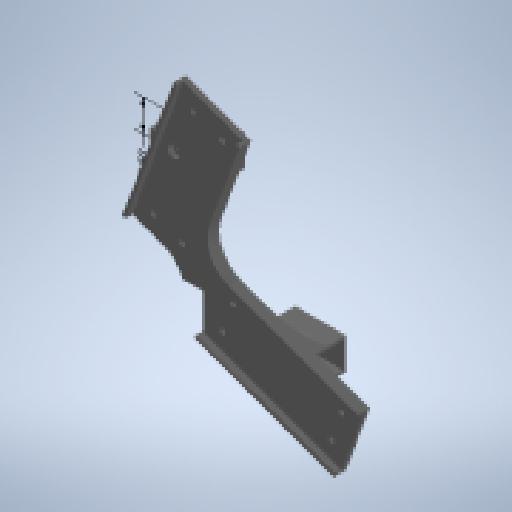
# Autodesk Inventor part: back_base
Saved by Autodesk Inventor 2026.1 (Build 301233020, 233B)
## iProperties
Created: 2026-02-04
Part Number: back_base
Material: 一般
Document SubType Name: Modeling
Designer: hibik
Density: 1 g/cm^3
Appearance: 既定
Author: hibik
Autodesk Inventor part; units mm, degrees
ref_plane "YZ Plane" through (0, 0, 0) normal (1, 0, 0) x (0, 1, 0)
ref_plane "XY Plane" through (0, 0, 0) normal (0, 0, 1) x (1, 0, 0)
sketch "スケッチ1" plane through (0, 0, 0) normal (1, 0, 0) x (0, 1, 0)
  line L0 (-7.75, -7.75) -> (7.75, -7.75)
  line L1 (7.75, -7.75) -> (7.75, 7.75)
  line L2 (7.75, 7.75) -> (-7.75, 7.75)
  line L3 (-7.75, 7.75) -> (-7.75, -7.75)
  line L4 (-7.75, -7.75) -> (7.75, 7.75) construction
  line L5 (7.75, -7.75) -> (-7.75, 7.75) construction
  line L6 (-9.25, 9.25) -> (9.25, 9.25)
  line L7 (9.25, 9.25) -> (9.25, -9.25)
  line L8 (9.25, -9.25) -> (-9.25, -9.25)
  line L9 (-9.25, -9.25) -> (-9.25, 9.25)
  line L10 (-9.25, 9.25) -> (9.25, -9.25) construction
  line L11 (9.25, 9.25) -> (-9.25, -9.25) construction
  point P0 (0, 0)
  dimension "d0" = 15.5
  dimension "d1" = 1.5
  constraints: 24 end point, 4 midpoint, 4 parallel, 3 perpendicular, 2 horizontal, 1 point on line
  measures "d0" distance of L2.end L1.end
  measures "d1" distance between parallel lines of L7 L1
extrude "押し出し1" add sketch "スケッチ1" along normal blind 30
sketch "スケッチ2" plane through (30, 9.25, -9.25) normal (0, 0, -1) x (-1, 0, 0)
  circle A0 centre (20, -9.25) radius 1.6
  line L0 (0, -18.5) -> (0, 0) projected
  point P0 (30, -9.25)
  dimension "d4" = 3.2
  dimension "d6" = 20
  constraints: 1 centre point, 1 horizontal alignment
  measures "d4" diameter of A0
  measures "d6" distance from line of L0 A0.centre
extrude "押し出し2" cut sketch "スケッチ2" against normal through all
sketch "スケッチ4" plane through (0, -9.25, 9.25) normal (0, 0, 1) x (1, 0, 0)
  line L0 (0, 18.5) -> (40, 18.5)
  line L1 (40, 18.5) -> (40, 0)
  line L2 (40, 0) -> (0, 0)
  line L3 (0, 0) -> (0, 18.5)
  circle A0 centre (10, 9.25) radius 1.6 projected
  point P0 (0, 9.25)
  dimension "d13" = 30
  constraints: 8 end point, 2 parallel, 1 horizontal, 1 perpendicular, 1 point on line
  measures "d13" distance from line of L1 A0.centre
extrude "押し出し4" add sketch "スケッチ4" along normal blind 7
sketch "スケッチ5" plane through (0, -9.25, 16.25) normal (0, 0, 1) x (1, 0, 0)
  line L0 (14.0213, 48.5) -> (52.5487, 34.4772)
  line L1 (52.5487, 34.4772) -> (-1.5009, -114.0228)
  line L2 (-1.5009, -114.0228) -> (-40.0283, -100)
  line L3 (-40.0283, -100) -> (14.0213, 48.5)
  line L4 (40, 0) -> (40, 18.5) projected
  line L5 (0, 0) -> (40, 0) projected
  line L6 (40, 18.5) -> (0, 18.5) projected
  line L7 (0, 18.5) -> (0, 0) projected
  point P0 (0, 9.25)
  point P1 (66.3687, 0)
  point P2 (3.1022, 18.5)
  dimension "d16" = 41
  dimension "d17" = 20
  dimension "d23" = 30
  dimension "d24" = 100
  constraints: 8 end point, 2 parallel, 1 perpendicular, 1 point on line
  measures "d16" distance between parallel lines of L1 L3
  measures "d17" angle of L4 L1
  measures "d23" distance from line of L0.start L6
  measures "d24" distance from line of L5 L2.end
extrude "押し出し5" add sketch "スケッチ5" against normal up to surface (7 mm away) contours L0 L1 L4 L6 L3 | L6 L4 L5 L7 L3 | L1 L2 L3 L7 L5
ref_plane "作業平面1" through (0, -82.75, 0) normal (0, 1, 0) x (-1, 0, 0)
ref_plane "作業平面2" through (0, -64.25, 0) normal (0, 1, 0) x (-1, 0, 0)
sketch "スケッチ13" plane through (0, -82.75, 0) normal (0, 1, 0) x (-1, 0, 0)
  line L0 (-60, 9.25) -> (-90, 9.25)
  line L1 (-90, 9.25) -> (-90, -9.25)
  line L2 (-90, -9.25) -> (-60, -9.25)
  line L3 (-60, -9.25) -> (-60, 9.25)
  line L4 (-3.1022, 9.25) -> (-30, 9.25) projected
  line L5 (0, -9.25) -> (-30, -9.25) projected
  line L6 (-30, -9.25) -> (-30, 9.25) projected
  point P0 (0, 0)
  dimension "d61" = 30
  dimension "d62" = 30
  constraints: 8 end point, 2 collinear, 2 parallel, 1 horizontal, 1 perpendicular
  measures "d61" distance between parallel lines of L3 L6
  measures "d62" distance of L0.start L0.end
extrude "押し出し11" add sketch "スケッチ13" along normal blind 18.5
sketch "スケッチ14" plane through (90, -82.75, 9.25) normal (1, 0, 0) x (0, 0, -1)
  line L0 (1.5, 17) -> (17, 17)
  line L1 (17, 17) -> (17, 1.5)
  line L2 (17, 1.5) -> (1.5, 1.5)
  line L3 (1.5, 1.5) -> (1.5, 17)
  line L4 (1.5, 17) -> (17, 1.5) construction
  line L5 (17, 17) -> (1.5, 1.5) construction
  line L6 (18.5, 0) -> (18.5, 18.5) projected
  line L7 (0, 18.5) -> (18.5, 18.5) projected
  point P0 (9.25, 82.75)
  point P1 (9.25, 9.25)
  point P2 (18.5, 9.25)
  point P3 (9.25, 18.5)
  dimension "d65" = 15.5
  constraints: 12 end point, 4 midpoint, 2 parallel, 2 perpendicular, 1 horizontal, 1 horizontal alignment, 1 vertical alignment
  measures "d65" distance of L1.end L2.end
extrude "押し出し12" cut sketch "スケッチ14" against normal through all
sketch "スケッチ15" plane through (0, -9.25, 16.25) normal (0, 0, 1) x (1, 0, 0)
  line L0 (15.9007, 47.816) -> (50.6693, 35.1612)
  line L1 (50.6693, 35.1612) -> (-3.3803, -113.3388)
  line L2 (-3.3803, -113.3388) -> (-38.1489, -100.684)
  line L3 (-38.1489, -100.684) -> (15.9007, 47.816)
  line L4 (14.0213, 48.5) -> (3.1022, 18.5) projected
  line L5 (52.5487, 34.4772) -> (14.0213, 48.5) projected
  line L6 (-40.0283, -100) -> (-1.5009, -114.0228) projected
  point P0 (0, 9.25)
  point P1 (33.285, 41.4886)
  dimension "d68" = 2
  constraints: 8 end point, 3 parallel, 2 midpoint, 1 collinear, 1 perpendicular, 1 point on line
  measures "d68" distance between parallel lines of L4 L3
extrude "押し出し13" cut sketch "スケッチ15" against normal blind 4
sketch "スケッチ16" plane through (0, -9.25, 12.25) normal (0, 0, 1) x (1, 0, 0)
  line L0 (14.0213, 48.5) -> (52.5487, 34.4772) projected
  line L1 (33.285, 41.4886) -> (-20.7646, -107.0114)
  line L2 (-3.3803, -113.3388) -> (-38.1489, -100.684) projected
  circle A0 centre (21.4075, 35.1698) radius 1.6
  circle A1 centre (38.322, 29.0135) radius 1.6
  circle A2 centre (9.7788, 3.2203) radius 1.6
  circle A3 centre (26.6933, -2.9361) radius 1.6
  circle A4 centre (-1.8498, -28.7293) radius 1.6
  circle A5 centre (15.0646, -34.8856) radius 1.6
  point P0 (0, 9.25)
  dimension "d71" = 3.2
  dimension "d72" = 9
  dimension "d73" = 10
  dimension "d76" = 34
  constraints: 6 centre point, 2 end point, 2 midpoint, 1 perpendicular, 10 other
  measures "d71" diameter of A0
  measures "d72" distance from line of L1 A0.centre
  measures "d73" distance from line of L0 A0.centre
  measures "d76" distance of A0.centre A2.centre
extrude "押し出し14" cut sketch "スケッチ16" against normal through all contours A0 | A1 | A4 | A5
sketch "スケッチ17" plane through (0, -9.25, 16.25) normal (0, 0, 1) x (1, 0, 0)
  line L0 (-40.0283, -100) -> (0, 9.9769) projected
  line L1 (-16.0765, -34.193) -> (60, -61.8825)
  line L2 (0, 9.9769) -> (-40.0283, -100) projected
  circle A0 centre (-1.8498, -28.7293) radius 1.6 projected
  line L3 (60, -73.5) -> (60, -55) projected
  line L4 (52.5487, 34.4772) -> (-1.5009, -114.0228) projected
  line L5 (22.4509, -48.2158) -> (28.1722, -32.4965)
  line L6 (28.1722, -32.4965) -> (90, -55)
  line L7 (90, -55) -> (84.2787, -70.7192)
  line L8 (84.2787, -70.7192) -> (22.4509, -48.2158)
  line L9 (60, -73.5) -> (90, -73.5) projected
  line L10 (90, -73.5) -> (90, -55) projected
  line L11 (60, -55) -> (90, -55) projected
  line L12 (60, -73.5) -> (60, -55) projected
  point P0 (0, 9.25)
  dimension "d83" = 10
  constraints: 10 end point, 5 point on line, 2 parallel, 2 perpendicular, 1 coincident
  measures "d83" distance from line of L1 A0.centre
extrude "押し出し15" add sketch "スケッチ17" against normal up to surface (7 mm away) contours L4 L6 L11 L3 L1 | L8 L7 L10 L9 L3 | L3 L11 L7 L8
sketch "スケッチ18" plane through (0, -9.25, 16.25) normal (0, 0, 1) x (1, 0, 0)
  circle A0 centre (15.0646, -34.8856) radius 1.6 projected
  circle A1 centre (38.322, 29.0135) radius 1.6 projected
  circle A2 centre (-1.8498, -28.7293) radius 1.6 projected
  circle A3 centre (21.4075, 35.1698) radius 1.6 projected
  line L0 (30, 18.5) -> (30, 0) projected
  line L1 (3.1022, 18.5) -> (30, 18.5) projected
  line L2 (3.1022, 18.5) -> (14.0213, 48.5) projected
  line L3 (14.0213, 48.5) -> (52.5487, 34.4772) projected
  line L4 (52.5487, 34.4772) -> (28.1722, -32.4965) projected
  line L5 (28.1722, -32.4965) -> (90, -55) projected
  line L6 (60, -55) -> (90, -55) projected
  line L7 (60, -61.8825) -> (60, -55) projected
  line L8 (60, -61.8825) -> (22.4509, -48.2158) projected
  line L9 (22.4509, -48.2158) -> (-1.5009, -114.0228) projected
  line L10 (-1.5009, -114.0228) -> (-40.0283, -100) projected
  line L11 (-40.0283, -100) -> (0, 9.9769) projected
  line L12 (0, 0) -> (0, 9.9769) projected
  line L13 (30, 0) -> (0, 0) projected
  line L14 (22.4509, -48.2158) -> (-16.0765, -34.193)
  line L15 (22.4509, -48.2158) -> (60, -61.8825) projected
  point P0 (0, 9.25)
  constraints: 2 end point, 1 collinear, 1 point on line
extrude "押し出し16" cut sketch "スケッチ18" against normal through all contours L14 L9 L10 L11
sketch "スケッチ19" plane through (0, -9.25, 16.25) normal (0, 0, 1) x (1, 0, 0)
  line L0 (28.1722, -32.4965) -> (14.1494, -71.0239)
  line L1 (14.1494, -71.0239) -> (108.1187, -105.2259)
  line L2 (108.1187, -105.2259) -> (122.1415, -66.6985)
  line L3 (122.1415, -66.6985) -> (28.1722, -32.4965)
  line L4 (90, -55) -> (28.1722, -32.4965) projected
  line L5 (28.1722, -32.4965) -> (52.5487, 34.4772) projected
  point P0 (0, 9.25)
  dimension "d88" = 41
  dimension "d89" = 100
  constraints: 8 end point, 3 point on line, 2 parallel, 1 perpendicular
  measures "d88" distance between parallel lines of L1 L3
  measures "d89" distance between parallel lines of L2 L0
extrude "押し出し17" add sketch "スケッチ19" against normal up to surface (7 mm away)
sketch "スケッチ20" plane through (0, -9.25, 16.25) normal (0, 0, 1) x (1, 0, 0)
  line L0 (122.1415, -66.6985) -> (108.1187, -105.2259) projected
  line L1 (121.4575, -68.5779) -> (108.8027, -103.3466)
  line L2 (108.8027, -103.3466) -> (26.1098, -73.2488)
  line L3 (26.1098, -73.2488) -> (38.7645, -38.4802)
  line L4 (38.7645, -38.4802) -> (121.4575, -68.5779)
  line L5 (122.1415, -66.6985) -> (28.1722, -32.4965) projected
  point P0 (0, 9.25)
  point P1 (115.1301, -85.9622)
  dimension "d92" = 2
  dimension "d93" = 88
  constraints: 8 end point, 2 midpoint, 2 parallel, 2 point on line, 1 perpendicular
  measures "d92" distance between parallel lines of L5 L4
  measures "d93" distance between parallel lines of L0 L3
extrude "押し出し18" cut sketch "スケッチ20" against normal blind 4
sketch "スケッチ21" plane through (0, -9.25, 12.25) normal (0, 0, 1) x (1, 0, 0)
  circle A0 centre (108.8113, -74.0848) radius 1.6
  circle A1 centre (102.655, -90.9993) radius 1.6
  line L0 (122.1415, -66.6985) -> (108.1187, -105.2259) projected
  line L1 (115.1301, -85.9622) -> (32.4371, -55.8645)
  line L2 (26.1098, -73.2488) -> (38.7645, -38.4802) projected
  circle A2 centre (76.8618, -62.4561) radius 1.6
  circle A3 centre (70.7054, -79.3706) radius 1.6
  circle A4 centre (44.9122, -50.8274) radius 1.6
  circle A5 centre (38.7559, -67.7419) radius 1.6
  point P0 (0, 9.25)
  dimension "d96" = 3.2
  dimension "d97" = 9
  dimension "d98" = 10
  dimension "d101" = 34
  constraints: 6 centre point, 2 end point, 2 midpoint, 10 other
  measures "d96" diameter of A0
  measures "d97" distance from line of L1 A0.centre
  measures "d98" distance from line of L0 A0.centre
  measures "d101" distance of A0.centre A2.centre
extrude "押し出し19" cut sketch "スケッチ21" against normal through all contours A0 | A1 | A4 | A5
fillet "フィレット1" radius 20 2 edges at (22.4509, -57.4658, 12.75) (28.1722, -41.7465, 12.75)
sketch "スケッチ22" plane through (0, -9.25, 12.25) normal (0, 0, 1) x (1, 0, 0)
  circle A0 centre (10, 9.25) radius 1.6 projected
  point P0 (0, 9.25)
extrude "押し出し20" cut sketch "スケッチ22" against normal through all
sketch "スケッチ23" plane through (0, -9.25, 12.25) normal (0, 0, 1) x (1, 0, 0)
  circle A0 centre (10, 9.25) radius 1.6 projected
  circle A1 centre (10, 9.25) radius 3.5
  point P0 (0, 9.25)
  dimension "d111" = 7
  constraints: 1 centre point, 1 coincident
  measures "d111" diameter of A1
extrude "押し出し21" cut sketch "スケッチ23" against normal blind 3
sketch "スケッチ24" plane through (0, -9.25, 9.25) normal (0, 0, -1) x (-1, 0, 0)
  line L0 (-60, -73.5) -> (-60, -55) projected
  line L1 (-60, -55) -> (-14.1494, -55)
  line L2 (-14.1494, -55) -> (-14.1494, -73.5)
  line L3 (-14.1494, -73.5) -> (-60, -73.5)
  line L4 (-60, -73.5) -> (-60, -55)
  line L5 (-14.1494, -55) -> (-27, -55)
  line L6 (-27, -55) -> (-27, -73.5)
  line L7 (-27, -73.5) -> (-14.1494, -73.5)
  line L8 (-14.1494, -73.5) -> (-14.1494, -55)
  circle A0 centre (-10, 9.25) radius 1.6 projected
  line L9 (-14.1494, -53) -> (-27, -53)
  line L10 (-27, -53) -> (-27, -75.7012)
  line L11 (-27, -75.7012) -> (-14.1494, -75.7012)
  line L12 (-14.1494, -75.7012) -> (-14.1494, -53)
  line L13 (-108.1187, -105.2259) -> (-14.1494, -71.0239) projected
  point P0 (0, 9.25)
  dimension "d114" = 17
  dimension "d115" = 2
  constraints: 24 end point, 6 parallel, 5 point on line, 3 horizontal, 3 perpendicular
  measures "d114" distance from line of A0.centre L6
  measures "d115" distance between parallel lines of L9 L1
extrude "押し出し22" cut sketch "スケッチ24" against normal through all contours L6 L1 L2 L13 L3 | L3 L13 L10 | L10 L9 L12 L1 | L13 L2 L3 | L3 L12 L11 L13
sketch "スケッチ25" plane through (0, -9.25, 16.25) normal (0, 0, 1) x (1, 0, 0)
  line L0 (38.7645, -38.4802) -> (121.4575, -68.5779) projected
  line L1 (50.6693, 35.1612) -> (18.5812, -53) projected
  line L2 (38.7645, -38.4802) -> (25.6088, -33.6919)
  line L3 (18.5812, -53) -> (27, -53) projected
  line L4 (27, -53) -> (27, -70.8029) projected
  line L5 (27, -70.8029) -> (38.7645, -38.4802) projected
  line L6 (38.7645, -38.4802) -> (121.4575, -68.5779) projected
  line L7 (121.4575, -68.5779) -> (122.1415, -66.6985) projected
  line L8 (122.1415, -66.6985) -> (46.9661, -39.3369) projected
  arc A0 (35.0126, -13.7027) -> (46.9661, -39.3369) centre (53.8065, -20.5431) ccw projected
  line L9 (35.0126, -13.7027) -> (52.5487, 34.4772) projected
  line L10 (52.5487, 34.4772) -> (50.6693, 35.1612) projected
  line L11 (50.6693, 35.1612) -> (18.5812, -53) projected
  point P0 (0, 9.25)
  point P1 (18.5812, -53)
  constraints: 2 end point, 1 perpendicular, 1 point on line
extrude "押し出し23" cut sketch "スケッチ25" against normal up to surface (4 mm away) contours L5 L4 L3 L1 L2
fillet "フィレット2" radius 10 4 edges at (16.5511, 9.25, 9.25) (15, -9.25, 9.25) (75, -82.75, 9.25) (75, -64.25, 9.25)
